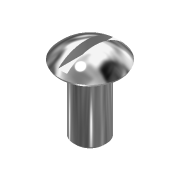
# Autodesk Inventor part: screw
Saved by Autodesk Inventor 2022 Beta2 (Build 260130000, 130) ContinuousBuild 0
## iProperties
Shininess: 86.0
Length Units: 11272
Angle Units: 11279
Time Units: 11290
Mass Units: 11286
Length Display Precision: 3
Angle Display Precision: 2
Created: 2001-07-20
Part Number: screw
Document SubType Name: Modeling
Designer: smithga
Density: 1 g/cm^3
Material: Generic
Appearance: Chrome - Polished
Density: 0.0
Volumn: 0.0
Area: 0.0
PropertySet Name: Model Information
Control State: 0
Master: False
Checked Out: False
Author: smithga
Autodesk Inventor part; units mm, degrees
ref_plane "YZ Plane" through (0, 0, 0) normal (1, 0, 0) x (0, 1, 0)
ref_plane "XZ Plane" through (0, 0, 0) normal (0, 1, 0) x (-1, 0, 0)
ref_plane "XY Plane" through (0, 0, 0) normal (0, 0, 1) x (1, 0, 0)
sketch "Sketch1" plane through (0, 0, 0) normal (0, 0, 1) x (1, 0, 0)
  line L0 (0, 7.9375) -> (0, 0)
  line L1 (0, 0) -> (1.5875, 0)
  line L2 (1.5875, 0) -> (1.5875, 6.3113)
  line L3 (1.5875, 6.3113) -> (3.175, 6.3113)
  arc A0 (3.175, 6.3113) -> (0, 7.9375) centre (0, 4.0249) ccw
  line L4 (-3.8487, 7.9375) -> (5.6755, 7.9375)
  dimension "d0" = 1.5875
  dimension "d1" = 1.5875
  dimension "d2" = 7.9375
  dimension "d10" = 3.9126
  constraints: 10 end point, 2 horizontal, 2 parallel, 2 point on circle, 2 vertical, 1 centre point, 1 perpendicular, 1 point on line, 1 tangent
  measures "d0" distance of L0.end L1.end
  measures "d1" distance of L2.end L3.end
  measures "d2" distance of L0.start L0.end
  measures "d10" radius of A0
revolve "Revolution1" add sketch "Sketch1" angle 360 about axis through (0, 7.9375, 0) along (0, -1, 0)
chamfer "Chamfer1" distance 0.254 angle 45 2 edges at (-1.5875, 0, 0) (-3.175, 6.3113, 0)
sketch "Sketch2" plane through (0, 0, 0) normal (0, 0, 1) x (1, 0, 0)
  line L0 (-0.4319, 9.1026) -> (0.4319, 9.1026)
  line L1 (0.4319, 9.1026) -> (0.4319, 6.8637)
  line L2 (0.4319, 6.8637) -> (-0.4319, 6.8637)
  line L3 (-0.4319, 6.8637) -> (-0.4319, 9.1026)
  line L4 (-1.5875, 6.3113) -> (-1.5875, 0.254) projected
  line L5 (1.5875, 6.3113) -> (1.5875, 0.254) projected
  dimension "d6" = 1.1556
  dimension "d7" = 1.1556
  constraints: 8 end point, 2 parallel, 1 horizontal, 1 perpendicular
  measures "d6" distance between parallel lines of L3 L4
  measures "d7" distance between parallel lines of L1 L5
extrude "Extrusion1" cut sketch "Sketch2" against normal mid plane 25.4
equation "\"d7\" = d6"
body "Solid1"
